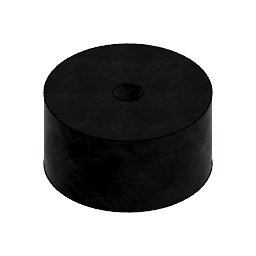
SHEX_004_hnbr_seal_expanded (Autodesk Fusion 360 design; units mm, degrees)
part number: 2026-05-30-09-03-59-943
Autodesk Fusion 360 part; units mm, degrees
sketch "Sketch1" plane through (0, 0, 0) normal (0, 0, 1) x (1, 0, 0)
  circle A0 centre (0, 0) radius 110.744
  circle A1 centre (0, 0) radius 19.685
extrude "Extrude1" add sketch "Sketch1" along normal blind 114.3
named bodies: "SHEX-004_hnbr_cup"
